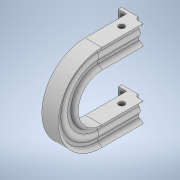
# Autodesk Inventor part: obejma2
Saved by Autodesk Inventor 2022 (Build 260153000, 153)
## iProperties
Created: 2022-05-17
Part Number: obejma2
Material: Ogólny
Document SubType Name: Modeling
Designer: Karle
Density: 1 g/cm^3
Appearance: Domyślna
Author: Karle
Autodesk Inventor part; units mm, degrees
ref_plane "YZ Plane" through (0, 0, 0) normal (1, 0, 0) x (0, 1, 0)
ref_plane "XZ Plane" through (0, 0, 0) normal (0, 1, 0) x (-1, 0, 0)
ref_plane "XY Plane" through (0, 0, 0) normal (0, 0, 1) x (1, 0, 0)
sketch "Szkic1" plane through (0, 0, 0) normal (0, 0, 1) x (1, 0, 0)
  line L0 (0, 0) -> (10, 0)
  line L1 (10, 12) -> (0, 12)
  arc A0 (10, 0) -> (7.5, 2) centre (7.165, -0.9812) ccw
  arc A1 (2.5, 2) -> (0, 0) centre (2.835, -0.9812) ccw
  arc A2 (7.5, 10) -> (10, 12) centre (7.165, 12.9812) ccw
  arc A3 (0, 12) -> (2.5, 10) centre (2.835, 12.9812) ccw
  arc A4 (7.5, 4) -> (7.5, 2) centre (8.8251, 3) ccw
  arc A5 (2.5, 2) -> (2.5, 4) centre (1.1749, 3) ccw
  arc A6 (7.5, 10) -> (7.5, 8) centre (8.8251, 9) ccw
  arc A7 (2.5, 8) -> (2.5, 10) centre (1.1749, 9) ccw
  arc A8 (7.5, 4) -> (7.5, 8) centre (5.2639, 6) ccw
  arc A9 (2.5, 8) -> (2.5, 4) centre (4.7361, 6) ccw
  line L2 (-1.9818, -14.25) -> (12.2979, -14.25)
  dimension "d0" = 10
  dimension "d5" = 3
  dimension "d7" = 3
  dimension "d10" = 3
  dimension "d11" = 3
  dimension "d12" = 3
  dimension "d13" = 3
  constraints: 21 point on circle, 10 centre point, 6 end point, 3 horizontal
  measures "d0" distance of L0.start L0.end
  measures "d5" radius of A0
  measures "d7" radius of A1
  measures "d10" radius of A2
  measures "d11" radius of A3
  measures "d12" radius of A8
  measures "d13" radius of A9
revolve "Obrót1" add sketch "Szkic1" angle 180 about axis through (-1.9818, -14.25, 0) along (1, 0, 0)
sketch "Szkic2" plane through (10, 0, 0) normal (0, 0, -1) x (-1, 0, 0)
  line L0 (10, 0) -> (0, 0) projected
  line L1 (0, 0) -> (10, 0)
  line L2 (0, 12) -> (10, 12) projected
  line L3 (0, 12) -> (10, 12)
  arc A0 (7.5, 10) -> (7.5, 8) centre (8.8251, 9) ccw projected
  line L4 (10, 12) -> (10, -40.5) projected
  arc A1 (2.5, 8) -> (2.5, 10) centre (1.1749, 9) ccw projected
  arc A2 (2.5, 8) -> (2.5, 4) centre (4.7361, 6) ccw projected
  arc A3 (2.5, 8) -> (2.5, 10) centre (1.175, 9) ccw
  arc A4 (7.5, 4) -> (7.5, 8) centre (5.2639, 6) ccw projected
  arc A5 (7.5, 10) -> (7.5, 8) centre (8.8251, 9) ccw
  arc A6 (7.5, 4) -> (7.5, 2) centre (8.8251, 3) ccw projected
  arc A7 (7.5, 4) -> (7.5, 8) centre (5.2639, 6) ccw
  line L5 (8.2639, 6) -> (8.2639, -34.5) projected
  arc A8 (2.5, 8) -> (2.5, 4) centre (4.7361, 6) ccw
  arc A9 (2.5, 2) -> (0, 0) centre (2.835, -0.9812) ccw projected
  arc A10 (2.5, 2) -> (2.5, 4) centre (1.1749, 3) ccw
  line L6 (2.835, 3) -> (2.835, -31.5) projected
  arc A11 (7.5, 4) -> (7.5, 2) centre (8.8251, 3) ccw
  arc A12 (2.5, 2) -> (0, 0) centre (2.835, -0.9812) ccw
  arc A13 (10, 0) -> (7.5, 2) centre (7.165, -0.9812) ccw projected
  arc A14 (10, 0) -> (7.5, 2) centre (7.165, -0.9812) ccw
  arc A15 (7.5, 10) -> (10, 12) centre (7.165, 12.9812) ccw
  arc A16 (7.5, 10) -> (10, 12) centre (7.165, 12.9812) ccw projected
  arc A17 (0, 12) -> (2.5, 10) centre (2.835, 12.9812) ccw
  arc A18 (0, 12) -> (2.5, 10) centre (2.835, 12.9812) ccw projected
  dimension "d16" = 1.66
  constraints: 20 point on circle, 10 centre point, 5 tangent, 4 end point, 3 concentric, 2 collinear
  measures "d16" radius of A3
extrude "Wyciągnięcie proste1" add sketch "Szkic2" along normal blind 25 contours L0 L5 A13 | L0 L6 A10 A2 A1 A17 L2 A15 A0 A4 A6 A13 L5 | L0 A9 A10 L6
sketch "Szkic3" plane through (10, -28.5, 0) normal (0, 0, -1) x (-1, 0, 0)
  line L0 (10, 0) -> (0, 0) projected
  line L1 (0, 0) -> (10, 0)
  arc A0 (2.5, -10) -> (0, -12) centre (2.835, -12.9812) ccw projected
  line L2 (0, -12) -> (10, -12) projected
  line L3 (0, -12) -> (10, -12)
  arc A1 (10, -12) -> (7.5, -10) centre (7.165, -12.9812) ccw projected
  arc A2 (10, -12) -> (7.5, -10) centre (7.165, -12.9812) ccw
  arc A3 (2.5, -10) -> (2.5, -8) centre (1.1749, -9) ccw projected
  arc A4 (2.5, -10) -> (0, -12) centre (2.835, -12.9812) ccw
  arc A5 (0, 0) -> (2.5, -2) centre (2.835, 0.9812) ccw projected
  arc A6 (2.5, -4) -> (2.5, -2) centre (1.1749, -3) ccw projected
  arc A7 (0, 0) -> (2.5, -2) centre (2.835, 0.9812) ccw
  line L4 (7.5, 30.5) -> (7.5, -2) projected
  arc A8 (7.5, -2) -> (10, 0) centre (7.165, 0.9812) ccw projected
  arc A9 (7.5, -2) -> (10, 0) centre (7.165, 0.9812) ccw
  arc A10 (7.5, -2) -> (7.5, -4) centre (8.8251, -3) ccw projected
  arc A11 (7.5, -2) -> (7.5, -4) centre (8.8251, -3) ccw
  arc A12 (2.5, -4) -> (2.5, -2) centre (1.1749, -3) ccw
  arc A13 (2.5, -4) -> (2.5, -8) centre (4.7361, -6) ccw projected
  arc A14 (2.5, -4) -> (2.5, -8) centre (4.7361, -6) ccw
  arc A15 (7.5, -8) -> (7.5, -4) centre (5.2639, -6) ccw projected
  arc A16 (7.5, -8) -> (7.5, -4) centre (5.2639, -6) ccw
  line L5 (7.5, 38.5) -> (7.5, -10) projected
  arc A17 (7.5, -8) -> (7.5, -10) centre (8.618, -9) ccw
  arc A18 (2.5, -10) -> (2.5, -8) centre (1.382, -9) ccw
  point P0 (10, 28.5)
  constraints: 20 point on circle, 10 centre point, 4 concentric, 4 end point, 3 tangent, 1 collinear, 1 horizontal
extrude "Wyciągnięcie proste2" add sketch "Szkic3" along normal blind 25 contours A8 L4 L0 | L4 A10 L5 A17 A1 L2 A0 A18 A13 A6 A5 L0 | A15 L5
sketch "Szkic4" plane through (0, 12, 0) normal (0, 1, 0) x (1, 0, 0)
  line L0 (0, 0) -> (10, 0) projected
  circle A0 centre (5, 17) radius 1.75
  dimension "d22" = 3.5
  constraints: 1 centre point
  measures "d22" diameter of A0
extrude "Wyciągnięcie proste3" cut sketch "Szkic4" against normal blind 250
sketch "Szkic5" plane through (0, 12, 0) normal (0, 1, 0) x (1, 0, 0)
  point P0 (0, 0)
sketch "Szkic6" plane through (10, 0, -25) normal (0, 0, -1) x (-1, 0, 0)
  line L0 (10, 12) -> (0, 12) projected
  line L1 (5, 12) -> (5, -40.5)
  line L2 (0, -40.5) -> (10, -40.5) projected
  line L3 (10, -28.5) -> (0, -28.5) projected
  line L4 (5, -28.5) -> (15, -28.5)
  line L5 (15, -28.5) -> (15, -40.5)
  line L6 (15, -40.5) -> (5, -40.5)
  line L7 (0, 0) -> (10, 0) projected
  line L8 (5, 0) -> (15, 0)
  line L9 (15, 0) -> (15, 12)
  line L10 (15, 12) -> (5, 12)
  line L11 (15, -34.5) -> (12, -34.5)
  line L12 (12, -34.5) -> (12, -30)
  line L13 (12, -34.5) -> (12, -39)
  line L14 (13.5, -30) -> (10.5, -30)
  line L15 (10.5, -30) -> (10.5, -39)
  line L16 (10.5, -39) -> (13.5, -39)
  line L17 (13.5, -39) -> (13.5, -30)
  dimension "d25" = 10
  dimension "d26" = 3
  dimension "d27" = 4.5
  dimension "d28" = 4.5
  dimension "d29" = 3
  constraints: 28 end point, 5 midpoint, 5 perpendicular, 4 equal length, 2 horizontal, 2 point on line, 1 vertical
  measures "d25" distance of L4.start L4.end
  measures "d26" distance of L11.start L11.end
  measures "d27" distance of L11.end L12.end
  measures "d28" distance of L11.end L13.end
  measures "d29" distance of L16.end L15.end
extrude "Wyciągnięcie proste4" add sketch "Szkic6" along normal blind 2 contours L3 L4 L5 L6 L2 L1
sketch "Szkic7" plane through (10, 0, -25) normal (0, 0, -1) x (-1, 0, 0)
  line L0 (0, 0) -> (10, 0) projected
  line L1 (5, 0) -> (5, 12)
  line L2 (10, 12) -> (0, 12) projected
  line L3 (5, 12) -> (15, 12)
  line L4 (15, 12) -> (15, 0)
  line L5 (15, 0) -> (5, 0)
  line L6 (15, 6) -> (12, 6)
  line L7 (12, 6) -> (12, 10.5)
  line L8 (12, 6) -> (12, 1.5)
  line L9 (13.5, 10.5) -> (10.5, 10.5)
  line L10 (10.5, 10.5) -> (10.5, 1.5)
  line L11 (10.5, 1.5) -> (13.5, 1.5)
  line L12 (13.5, 1.5) -> (13.5, 10.5)
  dimension "d32" = 10
  dimension "d33" = 3
  dimension "d34" = 4.5
  dimension "d35" = 4.5
  dimension "d36" = 3
  constraints: 22 end point, 4 perpendicular, 3 midpoint, 2 horizontal, 2 parallel, 2 vertical
  measures "d32" distance of L1.end L3.end
  measures "d33" distance of L6.start L6.end
  measures "d34" distance of L6.end L7.end
  measures "d35" distance of L6.end L8.end
  measures "d36" distance of L11.end L10.end
extrude "Wyciągnięcie proste5" add sketch "Szkic7" along normal blind 2
fillet "Zaokrąglenie1" radius 2 2 edges at (5, 6, -25) (5, -34.5, -25)
